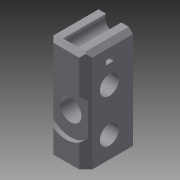
# Autodesk Inventor part: y-corners
Saved by Autodesk Inventor 2015 (Build 190159000, 159)
## iProperties
Created: 2015-04-27
Part Number: y-corners
Material: Generic
Document SubType Name: Modeling
Designer: mwang66
Density: 1 g/cm^3
Appearance: Default
Author: mwang66
Autodesk Inventor part; units mm, degrees
ref_plane "YZ Plane" through (0, 0, 0) normal (1, 0, 0) x (0, 1, 0)
ref_plane "XZ Plane" through (0, 0, 0) normal (0, 1, 0) x (-1, 0, 0)
ref_plane "XY Plane" through (0, 0, 0) normal (0, 0, 1) x (1, 0, 0)
sketch "Sketch1" plane through (0, 0, 0) normal (0, 0, 1) x (1, 0, 0)
  line L0 (9, -11) -> (-9, -11)
  line L1 (-9, -11) -> (-9, 11)
  line L2 (-9, 11) -> (9, 11)
  line L3 (9, 11) -> (9, -11)
  line L4 (9, -11) -> (-9, 11) construction
  line L5 (-9, -11) -> (9, 11) construction
  point P0 (0, 0)
  dimension "d0" = 18
  dimension "d1" = 22
  constraints: 12 end point, 2 midpoint, 2 parallel, 1 horizontal, 1 perpendicular
  measures "d0" distance of L1.end L2.end
  measures "d1" distance of L0.end L1.end
extrude "Extrusion1" add sketch "Sketch1" along normal blind 47
sketch "Sketch3" plane through (-9, 11, 0) normal (0, 1, 0) x (1, 0, 0)
  line L0 (18, -47) -> (0, -47) projected
  line L1 (9, 0) -> (9, -47) construction
  point P0 (9, -45.2)
  dimension "d31" = 1.8
  constraints: 2 end point, 1 midpoint, 1 point on line
  measures "d31" distance from line of L0 point (9, -45.2)
hole "Hole3" at (0, 11, 45.2) direction (0, -1, 0) diameter 8 depth 20
sketch "Sketch4" plane through (9, -11, 0) normal (1, 0, 0) x (0, 0, -1)
  line L0 (0, 11) -> (-47, 11) construction
  line L1 (-47, 0) -> (-47, 22) construction
  point P0 (-10, 11)
  point P1 (-30, 11)
  dimension "d33" = 17
  dimension "d42" = 20
  constraints: 2 end point, 2 point on line, 1 midpoint
  measures "d33" distance from line of L1 point (-30, 11)
  measures "d42" distance of point (-30, 11) point (-10, 11)
hole "Hole4" at (9, 0, 10) at (9, 0, 30) direction (-1, 0, 0) diameter 8.8 end through all
chamfer "Chamfer1" distance 3 angle 45 1 edges at (9, -11, 23.5)
chamfer "Chamfer2" distance 3 angle 45 1 edges at (-9, -11, 23.5)
chamfer "Chamfer3" distance 2 angle 45 1 edges at (0, -11, 47)
chamfer "Chamfer4" distance 2 angle 45 1 edges at (9, 1.5, 47)
chamfer "Chamfer5" distance 2 angle 45 1 edges at (-9, 1.5, 47)
sketch "Sketch6" plane through (-6, -11, 0) normal (0, -1, 0) x (1, 0, 0)
  line L0 (0, 45) -> (12, 45) construction
  line L1 (6, 45) -> (6, 0) construction
  line L2 (12, 0) -> (0, 0) construction
  point P0 (6, 20)
  dimension "d67" = 20
  constraints: 2 end point, 1 midpoint, 1 point on line, 1 vertical
  measures "d67" distance from line of L2 point (6, 20)
hole "Hole5" at (0, -11, 20) direction (0, 1, 0) diameter 10 end through all counterbore diameter 22 counterbore depth 2
sketch "Sketch7" plane through (-9, -8, 0) normal (-1, 0, 0) x (0, 0, 1)
  line L0 (38.675, 9.987) -> (40.675, 9.987)
  line L1 (40.675, 9.987) -> (40.675, 6.487)
  line L2 (40.675, 6.487) -> (38.675, 6.487)
  line L3 (38.675, 6.487) -> (38.675, 9.987)
  line L4 (47, -1) -> (47, 19) projected
  line L5 (29.2195, -3) -> (45, -3) projected
  point P0 (0, 8)
  dimension "d75" = 2
  dimension "d76" = 3.5
  dimension "d77" = 6.325
  dimension "d78" = 9.487
  constraints: 8 end point, 2 parallel, 1 horizontal, 1 perpendicular
  measures "d75" distance of L0.start L0.end
  measures "d76" distance of L2.end L0.start
  measures "d77" distance between parallel lines of L4 L1
  measures "d78" distance between parallel lines of L5 L2
extrude "Extrusion4" cut sketch "Sketch7" against normal through all
sketch "Sketch8" plane through (0, 0, 47) normal (0, 0, 1) x (1, 0, 0)
  line L0 (1, 1.5) -> (-1, 1.5)
  line L1 (-1, 1.5) -> (-1, -2)
  line L2 (-1, -2) -> (1, -2)
  line L3 (1, -2) -> (1, 1.5)
  line L4 (-6, -11) -> (6, -11) projected
  line L5 (-7, -9) -> (-7, 11) projected
  line L6 (-9, 11) -> (-9, -8) projected
  point P0 (0, 0)
  dimension "d81" = 2
  dimension "d82" = 3.5
  dimension "d83" = 9
  dimension "d85" = 8
  constraints: 8 end point, 2 parallel, 1 horizontal, 1 perpendicular
  measures "d81" distance of L0.start L0.end
  measures "d82" distance of L2.end L0.start
  measures "d83" distance between parallel lines of L4 L2
  measures "d85" distance between parallel lines of L6 L1
extrude "Extrusion5" cut sketch "Sketch8" against normal up to surface (8.325 mm away)
body "Solid1"
